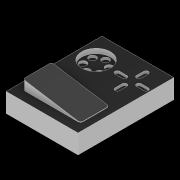
# Autodesk Inventor part: Tarefa 4
Saved by Autodesk Inventor 2020 (Build 240168000, 168)
## iProperties
Created: 2021-01-20
Part Number: Tarefa 4
Material: Glass
Document SubType Name: Modeling
Designer: Pedro Barriviera
Density: 2.18 g/cm^3
Appearance: Chrome - Polished
Author: Pedro Barriviera
Autodesk Inventor part; units mm, degrees
ref_plane "YZ Plane" through (0, 0, 0) normal (1, 0, 0) x (0, 1, 0)
ref_plane "XZ Plane" through (0, 0, 0) normal (0, 1, 0) x (-1, 0, 0)
sketch "Sketch1" plane through (0, 0, 0) normal (0, 1, 0) x (-1, 0, 0)
  line L0 (75, -100) -> (-75, -100)
  line L1 (-75, -100) -> (-75, 100)
  line L2 (-75, 100) -> (75, 100)
  line L3 (75, 100) -> (75, -100)
  line L4 (75, -100) -> (-75, 100) construction
  line L5 (-75, -100) -> (75, 100) construction
  line L6 (55, 80) -> (-55, 80)
  line L7 (-60, 75) -> (-60, 25)
  line L8 (-55, 20) -> (55, 20)
  line L9 (60, 25) -> (60, 75)
  line L10 (60, 80) -> (-60, 20) construction
  line L11 (-60, 80) -> (60, 20) construction
  circle A0 centre (38, -50.6667) radius 30
  circle A1 centre (38, -70.6667) radius 7.5
  circle A2 centre (55.3205, -60.6667) radius 7.5
  circle A3 centre (55.3205, -40.6667) radius 7.5
  circle A4 centre (38, -30.6667) radius 7.5
  circle A5 centre (20.6795, -40.6667) radius 7.5
  circle A6 centre (20.6795, -60.6667) radius 7.5
  arc A7 (55, 20) -> (60, 25) centre (55, 25) ccw
  arc A8 (60, 75) -> (55, 80) centre (55, 75) ccw
  arc A9 (-55, 80) -> (-60, 75) centre (-55, 75) ccw
  arc A10 (-60, 25) -> (-55, 20) centre (-55, 25) ccw
  arc A11 (-42, -64.1421) -> (-41.9301, -64.1667) centre (-37, -50) ccw
  arc A12 (-22, -45) -> (-22, -55) centre (-22, -50) ccw
  arc A13 (-7, -55) -> (-7, -45) centre (-7, -50) ccw
  line L12 (-7, -45) -> (-22, -45)
  line L13 (-7, -55) -> (-22, -55)
  line L14 (-42, -20) -> (-42, -35)
  arc A14 (-42, -35) -> (-32, -35) centre (-37, -35) ccw
  line L15 (-32, -20) -> (-32, -35)
  arc A15 (-32, -20) -> (-42, -20) centre (-37, -20) ccw
  line L16 (-67, -55) -> (-52, -55)
  arc A16 (-52, -55) -> (-52, -45) centre (-52, -50) ccw
  line L17 (-67, -45) -> (-52, -45)
  arc A17 (-67, -45) -> (-67, -55) centre (-67, -50) ccw
  line L18 (-32, -80) -> (-32, -65)
  arc A18 (-32, -65) -> (-42, -65) centre (-37, -65) ccw
  line L19 (-42, -80) -> (-42, -65)
  arc A19 (-42, -80) -> (-32, -80) centre (-37, -80) ccw
  point P0 (0, 0)
  point P1 (0, 50)
  dimension "d0" = 150
  dimension "d1" = 200
  dimension "d2" = 50
  dimension "d3" = 75
  dimension "d4" = 60
  dimension "d5" = 120
  dimension "d29" = 15
  dimension "d30" = 20
  dimension "d33" = 360
  dimension "d35" = 5
  dimension "d36" = 5
  dimension "d37" = 30
  dimension "d38" = 100
  dimension "d39" = 38
  dimension "d42" = 15
  dimension "d45" = 360
  dimension "d47" = 75
  dimension "d62" = 60
  dimension "d63" = 5
  dimension "d64" = 5
  constraints: 40 end point, 28 point on circle, 20 centre point, 12 tangent, 10 point on line, 8 coincident, 4 midpoint, 4 parallel, 2 equal radius, 2 horizontal, 2 horizontal alignment, 2 perpendicular, 1 vertical alignment, 56 other
  measures "d0" distance of L1.end L2.end
  measures "d1" distance of L0.end L1.end
  measures "d2" distance from line of L2 point (0, 50)
  measures "d3" distance from line of L1 point (0, 50)
  measures "d4" distance of L11.end L10.start
  measures "d5" distance of L10.end L11.end
  measures "d29" diameter of A1
  measures "d30" distance of A0.centre A1.centre
  measures "d35" radius of A7
  measures "d36" radius of A8
  measures "d37" diameter of A11
  measures "d38" vertical distance of point (0, 50) A11.centre
  measures "d39" distance from line of L1 A11.centre
  measures "d42" distance of A12.centre A13.centre
  measures "d47" horizontal distance of A11.centre A0.centre
  measures "d62" diameter of A0
  measures "d63" radius of A13
  measures "d64" radius of A12
extrude "Extrusion1" add sketch "Sketch1" along normal blind 40 contours L0 L1 L2 L3
extrude "Extrusion2" add sketch "Sketch1" along normal blind 60 contours A8 L9 A7 L8 A10 L7 A9 L6
extrude "Extrusion3" add sketch "Sketch1" along normal blind 30 contours A0
extrude "Extrusion4" add sketch "Sketch1" along normal blind 35 contours L12 A13 L13 A12 | A15 L15 A14 L14 | A17 L17 A16 L16 | A19 L19 A18 L18
extrude "Extrusion5" add sketch "Sketch1" along normal blind 25 contours A1 | A2 | A3 | A4 | A5 | A6
ref_plane "Work Plane1" through (-55, 40, 80) normal (0, 0, 1) x (1, 0, 0)
sketch "Sketch2" plane through (-55, 40, 80) normal (0, 0, 1) x (1, 0, 0)
  line L0 (-5, 0) -> (-5, 20) projected
  line L1 (-5, 20) -> (121.275, 0)
  line L2 (-5, 20) -> (122.8491, 20) construction
  line L3 (121.275, 0) -> (121.275, 40.187)
  line L4 (122, 0) -> (127, 0) projected
  line L5 (121.275, 40.187) -> (-5, 40.187)
  line L6 (-5, 40.187) -> (-5, 20)
  point P0 (55, -40)
  dimension "d59" = 9
  constraints: 10 end point, 2 perpendicular, 1 equal length, 1 horizontal
  measures "d59" angle of L1 L2
extrude "Extrusion6" cut sketch "Sketch2" against normal through all
body "Solid1"
